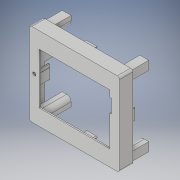
# Autodesk Inventor part: case_top
Saved by Autodesk Inventor 2019 (Build 230136000, 136)
## iProperties
Created: 2019-03-26
Part Number: case_top
Material: Generic
Document SubType Name: Modeling
Designer: janza
Density: 1 g/cm^3
Appearance: Default
Author: janza
## iProperties of the stored document case_top_3DPrint.ipt
Created: 2019-03-30
Part Number: case_top_3DPrint
Material: Generic
Document SubType Name: Modeling
Designer: janza
Density: 1 g/cm^3
Appearance: Default
Author: janza
Autodesk Inventor part; units mm, degrees
ref_plane "YZ Plane" through (0, 0, 0) normal (1, 0, 0) x (0, 1, 0)
ref_plane "XZ Plane" through (0, 0, 0) normal (0, 1, 0) x (-1, 0, 0)
ref_plane "XY Plane" through (0, 0, 0) normal (0, 0, 1) x (1, 0, 0)
sketch "vrsek" plane through (0, 0, 0) normal (0, 0, 1) x (1, 0, 0)
  line L0 (0, 0) -> (78.5, 0)
  line L1 (78.5, 0) -> (78.5, 72)
  line L2 (78.5, 72) -> (0, 72)
  line L3 (0, 72) -> (0, 0)
  dimension "d0" = 78.5
  dimension "d1" = 72
  constraints: 8 end point, 2 parallel, 1 horizontal, 1 perpendicular
  measures "d0" distance of L2.end L1.end
  measures "d1" distance of L1.end L0.end
extrude "Extrusion1" add sketch "vrsek" along normal blind 1.2 and the other way blind 0.4
sketch "displej_vyrez" plane through (0, 0, 1.2) normal (0, 0, 1) x (1, 0, 0)
  line L0 (0, 72) -> (0, 0) projected
  line L1 (78.5, 0) -> (78.5, 72) projected
  line L2 (0, 36) -> (7, 36)
  line L3 (7, 36) -> (7, 59.15)
  line L4 (7, 59.15) -> (71.2, 59.15)
  line L5 (71.2, 59.15) -> (71.2, 53.35)
  line L6 (71.2, 53.35) -> (72.7, 53.35)
  line L7 (72.7, 53.35) -> (72.7, 40.95)
  line L8 (72.7, 40.95) -> (71.2, 40.95)
  line L9 (7, 36) -> (7, 12.85)
  line L10 (7, 12.85) -> (71.2, 12.85)
  line L11 (71.2, 12.85) -> (71.2, 40.95)
  line L12 (0, 0) -> (78.5, 0) projected
  dimension "d4" = 7
  dimension "d5" = 23.15
  dimension "d6" = 64.2
  dimension "d7" = 5.8
  dimension "d8" = 1.5
  dimension "d9" = 12.4
  dimension "d10" = 1.5
  dimension "d11" = 23.15
  dimension "d12" = 36
  constraints: 20 end point, 6 perpendicular, 1 horizontal, 1 midpoint, 1 parallel, 1 point on line, 1 vertical
  measures "d4" distance of L2.start L2.end
  measures "d5" distance of L2.end L3.end
  measures "d6" distance of L3.end L4.end
  measures "d7" distance of L4.end L5.end
  measures "d8" distance of L5.end L6.end
  measures "d9" distance of L6.end L7.end
  measures "d10" distance of L7.end L8.end
  measures "d11" distance of L2.end L9.end
  measures "d12" distance between parallel lines of L12 L2
extrude "Extrusion2" cut sketch "displej_vyrez" against normal blind 3
sketch "resetTL_zarez_vedeni" plane through (0, 0, 1.2) normal (0, 0, 1) x (1, 0, 0)
  line L0 (0.5, 40.85) -> (5, 40.85)
  line L1 (5, 40.85) -> (5, 33.85)
  line L2 (5, 33.85) -> (0.5, 33.85)
  line L3 (0.5, 33.85) -> (0.5, 40.85)
  line L4 (0, 0) -> (78.5, 0) projected
  line L5 (7, 12.85) -> (7, 59.15) projected
  line L6 (71.2, 12.85) -> (7, 12.85) projected
  dimension "d15" = 4.5
  dimension "d16" = 7
  dimension "d19" = 2
  dimension "d20" = 21
  constraints: 8 end point, 2 parallel, 1 horizontal, 1 perpendicular
  measures "d15" distance of L1.end L2.end
  measures "d16" distance of L0.end L1.end
  measures "d19" distance between parallel lines of L5 L1
  measures "d20" distance between parallel lines of L6 L2
sketch "resetTL_vnitrek_vybrani" plane through (0, 0, -0.4) normal (0, 0, -1) x (-1, 0, 0)
  line L0 (-5, 33.85) -> (-0.8, 33.85)
  line L1 (-5, 40.85) -> (-5, 33.85)
  line L2 (-0.8, 40.85) -> (-5, 40.85)
  line L3 (-0.8, 33.85) -> (-0.8, 40.85)
  line L4 (0, 0) -> (0, 72) projected
  line L5 (0, 72) -> (0, 0) projected
  line L6 (0, 72) -> (-78.5, 72) projected
  point P0 (-0.8, 37.35)
  dimension "d106" = 31.15
  dimension "d107" = 4.2
  dimension "d108" = 7
  dimension "d109" = 0.8
  constraints: 8 end point, 1 midpoint
  measures "d106" distance between parallel lines of L6 L2
  measures "d107" distance of L2.start L1.start
  measures "d108" distance of L1.start L0.start
  measures "d109" distance between parallel lines of L4 L3
extrude "Extrusion3" cut sketch "resetTL_vnitrek_vybrani" against normal blind 0.9
sketch "resetTL_dira" plane through (0, 0, 0.5) normal (0, 0, -1) x (-1, 0, 0)
  line L0 (-5, 33.85) -> (-5, 40.85)
  circle A0 centre (-2.743122, 37.35) radius 1.5
  point P0 (0, 0)
  dimension "d23" = 3
  constraints: 1 centre point
  measures "d23" diameter of A0
extrude "Extrusion4" cut sketch "resetTL_dira" against normal blind 2
sketch "spojeni_srouby" plane through (0, 0, -0.4) normal (0, 0, -1) x (-1, 0, 0)
  line L0 (-8, 68) -> (-8, 72)
  line L1 (-4, 72) -> (0, 72)
  line L2 (-8, 72) -> (0, 72)
  line L3 (0, 72) -> (0, 71.785113)
  line L4 (0, 72) -> (0, 0)
  line L5 (0, 0) -> (0, 36)
  line L6 (-8, 4) -> (-8, 0)
  line L7 (-4, 0) -> (0, 0)
  line L8 (-8, 0) -> (0, 0)
  line L9 (0, 0) -> (0, 0.214887)
  line L10 (0, 0) -> (0, 72)
  line L11 (-70.5, 68) -> (-70.5, 72)
  line L12 (-74.5, 72) -> (-78.5, 72)
  line L13 (-70.5, 72) -> (-78.5, 72)
  line L14 (-78.5, 72) -> (-78.5, 71.785113)
  line L15 (-70.5, 4) -> (-70.5, 0)
  line L16 (-74.5, 0) -> (-78.5, 0)
  line L17 (-70.5, 0) -> (-78.5, 0)
  line L18 (-78.5, 0) -> (-78.5, 0.214887)
  line L19 (-78.5, 72) -> (-78.5, 72)
  line L20 (-78.5, 0) -> (-78.5, 0)
  line L21 (-78.5, 0) -> (-70.5, 0)
  line L22 (-74.5, 64) -> (-78.5, 64)
  line L23 (-78.5, 64) -> (-78.5, 72)
  arc A0 (-74.5, 64) -> (-70.5, 68) centre (-74.5, 68) ccw
  line L24 (-74.5, 8) -> (-78.5, 8)
  arc A1 (-70.5, 4) -> (-74.5, 8) centre (-74.5, 4) ccw
  line L25 (-4, 8) -> (0, 8)
  arc A2 (-4, 8) -> (-8, 4) centre (-4, 4) ccw
  line L26 (-4, 64) -> (0, 64)
  arc A3 (-8, 68) -> (-4, 64) centre (-4, 68) ccw
  line L27 (0, 72) -> (0, 56.55)
  line L28 (0, 72) -> (0, 64)
  line L29 (0, 8) -> (0, 0)
  line L30 (-78.5, 0) -> (-78.5, 8)
  line L31 (-78.5, 64) -> (-78.5, 72)
  line L32 (-70.5, 72) -> (-78.5, 72)
  line L33 (0, 72) -> (-8, 72)
  constraints: 68 end point, 8 point on circle, 5 perpendicular, 4 centre point, 4 tangent, 3 collinear, 2 point on line, 2 vertical, 1 midpoint
extrude "Extrusion7" add sketch "spojeni_srouby" along normal blind 26.5
sketch "diry_zavitova_vlozka" plane through (0, 0, -26.9) normal (0, 0, -1) x (-1, 0, 0)
  arc A0 (-70.5, 4) -> (-74.5, 8) centre (-74.5, 4) ccw projected
  arc A1 (-4, 8) -> (-8, 4) centre (-4, 4) ccw projected
  arc A2 (-8, 68) -> (-4, 64) centre (-4, 68) ccw projected
  arc A3 (-74.5, 64) -> (-70.5, 68) centre (-74.5, 68) ccw projected
  point P0 (0, 0)
  constraints: 4 coincident
hole "Hole1" at (74.5, 4, -26.9) at (4, 4, -26.9) at (4, 68, -26.9) at (74.5, 68, -26.9) direction (0, 0, 1) diameter 3.3 depth 12 countersink diameter 3.75 countersink angle 10
sketch "Sketch10" plane through (0, 0, -0.4) normal (0, 0, -1) x (-1, 0, 0)
  line L0 (-71.2, 59.15) -> (-7, 59.15) projected
  line L1 (-7, 59.15) -> (-7, 12.85) projected
  line L2 (-7, 12.85) -> (-71.2, 12.85) projected
  line L3 (-71.2, 12.85) -> (-71.2, 40.95) projected
  line L4 (-71.2, 40.95) -> (-72.7, 40.95) projected
  line L5 (-72.7, 40.95) -> (-72.7, 53.35) projected
  line L6 (-72.7, 53.35) -> (-71.2, 53.35) projected
  line L7 (-70.5, 0) -> (-8, 0) projected
  line L8 (-8, 0) -> (-8, 4) projected
  arc A0 (-4, 8) -> (-8, 4) centre (-4, 4) ccw projected
  line L9 (-4, 8) -> (0, 8) projected
  line L10 (0, 8) -> (0, 64) projected
  line L11 (0, 64) -> (-4, 64) projected
  arc A1 (-8, 68) -> (-4, 64) centre (-4, 68) ccw projected
  line L12 (-8, 68) -> (-8, 72) projected
  line L13 (-8, 72) -> (-70.5, 72) projected
  line L14 (-78.5, 64) -> (-78.5, 8) projected
  line L15 (-0.8, 40.85) -> (-0.8, 33.85) projected
  line L16 (-0.8, 33.85) -> (-5, 33.85) projected
  line L17 (-5, 33.85) -> (-5, 40.85) projected
  line L18 (-5, 40.85) -> (-0.8, 40.85) projected
  line L19 (-7, 12.85) -> (-71.2, 12.85) projected
  line L20 (-71.2, 12.85) -> (-71.2, 40.95) projected
  line L21 (-71.2, 40.95) -> (-72.7, 40.95) projected
  line L22 (-72.7, 40.95) -> (-72.7, 53.35) projected
  line L23 (-72.7, 53.35) -> (-71.2, 53.35) projected
  line L24 (-71.2, 53.35) -> (-71.2, 59.15) projected
  line L25 (-71.2, 59.15) -> (-7, 59.15) projected
  line L26 (-7, 59.15) -> (-7, 12.85) projected
  line L27 (-73.7, 61.65) -> (-73.7, 55.85)
  line L28 (-73.7, 55.85) -> (-75.2, 55.85)
  line L29 (-75.2, 55.85) -> (-75.2, 38.45)
  line L30 (-75.2, 38.45) -> (-73.7, 38.45)
  line L31 (-73.7, 38.45) -> (-73.7, 10.35)
  line L32 (-73.7, 10.35) -> (-4.5, 10.35)
  line L33 (-4.5, 10.35) -> (-4.5, 61.65)
  line L34 (-4.5, 61.65) -> (-73.7, 61.65)
  line L35 (-70.5, 4) -> (-70.5, 0) projected
  line L36 (-70.5, 72) -> (-70.5, 68) projected
  arc A2 (-74.5, 64) -> (-70.5, 68) centre (-74.5, 68) ccw projected
  line L37 (-74.5, 64) -> (-78.5, 64) projected
  line L38 (-78.5, 8) -> (-74.5, 8) projected
  arc A3 (-70.5, 4) -> (-74.5, 8) centre (-74.5, 4) ccw projected
  point P0 (0, 0)
  dimension "d58" = 2.5
  constraints: 16 end point, 7 other
  measures "d58" distance between parallel lines of L24 L27
extrude "Extrusion8" cut sketch "Sketch10" against normal blind 0.4 contours L33 L16 L17 L18 | L18 L17 L16 L33 L32 L31 L30 L29 L28 L27 L34
sketch "dira_RJ45" plane through (0, 0, -0.4) normal (0, 0, -1) x (-1, 0, 0)
  line L0 (1.6, 39.75) -> (0, 39.75)
  line L1 (0, 39.75) -> (0, 56.55)
  line L2 (0, 56.55) -> (1.6, 56.55)
  line L3 (1.6, 56.55) -> (1.6, 39.75)
  line L4 (-70.5, 0) -> (-8, 0) projected
  line L5 (0, 8) -> (0, 64) projected
  line L6 (0, 72) -> (-8, 72) projected
  point P0 (0, 0)
  point P1 (-78.5, 0)
  dimension "d61" = 1.6
  dimension "d62" = 16.8
  dimension "d64" = 0
  dimension "d74" = 15.45
  constraints: 8 end point, 2 parallel, 1 horizontal, 1 perpendicular
  measures "d61" distance of L1.end L2.end
  measures "d62" distance of L0.end L1.end
  measures "d64" distance between parallel lines of L5 L1
  measures "d74" distance between parallel lines of L6 L2
extrude "Extrusion9" add sketch "dira_RJ45" along normal blind 17.3 and the other way blind 1.6
sketch "Sketch12" plane through (0, 0, -0.4) normal (0, 0, -1) x (-1, 0, 0)
  line L0 (0, 56.55) -> (0, 64) projected
  line L1 (0, 64) -> (0, 72) projected
  line L2 (0, 72) -> (-8, 72) projected
  line L3 (-8, 72) -> (-70.5, 72) projected
  line L4 (-70.5, 72) -> (-78.5, 72) projected
  line L5 (-78.5, 72) -> (-78.5, 64) projected
  line L6 (-78.5, 64) -> (-78.5, 8) projected
  line L7 (-92, 8) -> (-92, 0) projected
  line L8 (-78.5, 0) -> (-70.5, 0) projected
  line L9 (-70.5, 0) -> (-8, 0) projected
  line L10 (-8, 0) -> (0, 0) projected
  line L11 (0, 0) -> (0, 8) projected
  line L12 (0, 8) -> (0, 39.75) projected
  line L13 (1.6, 56.55) -> (1.6, 63)
  line L14 (1.6, 63) -> (1.6, 73.6)
  line L15 (1.6, 73.6) -> (-8, 73.6)
  line L16 (-8, 73.6) -> (-80.1, 73.6)
  line L17 (-80.1, 73.6) -> (-80.1, 64)
  line L18 (-80.1, 64) -> (-80.1, 8)
  line L19 (-80.1, -1.6) -> (-8, -1.6)
  line L20 (-8, -1.6) -> (1.6, -1.6)
  line L21 (1.6, -1.6) -> (1.6, 7)
  line L22 (1.6, 7) -> (1.6, 39.75)
  line L23 (1.6, 56.55) -> (0, 56.55) projected
  line L24 (0, 56.55) -> (1.6, 56.55)
  line L25 (0, 39.75) -> (0, 56.55) projected
  line L26 (1.6, 39.75) -> (0, 39.75)
  line L27 (-80.1, 8) -> (-80.1, -1.6)
  constraints: 26 end point, 1 collinear, 1 horizontal, 1 perpendicular, 5 other
sketch "Sketch12 outline for Extrusion10" plane through (0, 0, -0.4) normal (0, 0, -1) x (-1, 0, 0)
  line L0 (0, 8) -> (0, 0)
  line L1 (0, 39.75) -> (0, 8)
  line L2 (1.6, 39.75) -> (0, 39.75)
  line L3 (1.6, 7) -> (1.6, 39.75)
  line L4 (1.6, -1.6) -> (1.6, 7)
  line L5 (-8, -1.6) -> (1.6, -1.6)
  line L6 (-80.1, -1.6) -> (-8, -1.6)
  line L7 (-80.1, 8) -> (-80.1, -1.6)
  line L8 (-80.1, 64) -> (-80.1, 8)
  line L9 (-80.1, 73.6) -> (-80.1, 64)
  line L10 (-8, 73.6) -> (-80.1, 73.6)
  line L11 (1.6, 73.6) -> (-8, 73.6)
  line L12 (1.6, 63) -> (1.6, 73.6)
  line L13 (1.6, 56.55) -> (1.6, 63)
  line L14 (0, 56.55) -> (1.6, 56.55)
  line L15 (0, 64) -> (0, 56.55)
  line L16 (0, 72) -> (0, 64)
  line L17 (-8, 72) -> (0, 72)
  line L18 (-70.5, 72) -> (-8, 72)
  line L19 (-78.5, 72) -> (-70.5, 72)
  line L20 (-78.5, 64) -> (-78.5, 72)
  line L21 (-78.5, 8) -> (-78.5, 64)
  line L22 (-78.5, 0) -> (-78.5, 8)
  line L23 (-70.5, 0) -> (-78.5, 0)
  line L24 (-8, 0) -> (-70.5, 0)
  line L25 (0, 0) -> (-8, 0)
extrude "Extrusion10" add sketch "Sketch12 outline for Extrusion10" along normal blind 10.5 and the other way blind 1.6
fillet "Fillet1" radius 2 4 edges at (-1.6, 73.6, -4.85) (-1.6, -1.6, -4.85) (80.1, 73.6, -4.85) (80.1, -1.6, -4.85)
sketch "Sketch13" plane through (0, 0, -0.4) normal (0, 0, -1) x (-1, 0, 0)
  line L0 (-1.2, 33.75) -> (-1.2, 24.65)
  line L1 (-0.4, 23.85) -> (0, 23.85)
  line L2 (0, 23.85) -> (0, 36.75)
  line L3 (0, 8) -> (0, 64) projected
  line L4 (0, 36.75) -> (-0.4, 36.75)
  line L5 (-0.8, 36.35) -> (-0.8, 33.95)
  line L6 (-0.8, 33.85) -> (-4.5, 33.85) projected
  line L7 (-0.9, 33.85) -> (-1.1, 33.85)
  arc A0 (-0.4, 36.75) -> (-0.8, 36.35) centre (-0.4, 36.35) ccw
  line L8 (-35.05, 1.2) -> (-43.45, 1.2)
  line L9 (-44.25, 0.4) -> (-44.25, 0)
  line L10 (-44.25, 0) -> (-34.25, 0)
  line L11 (-34.25, 0) -> (-34.25, 0.4)
  line L12 (-70.5, 0) -> (-8, 0) projected
  arc A1 (-1.2, 24.65) -> (-0.4, 23.85) centre (-0.4, 24.65) ccw
  line L13 (-34.25, 72) -> (-44.25, 72)
  line L14 (-44.25, 72) -> (-44.25, 71.6)
  line L15 (-43.45, 70.8) -> (-35.05, 70.8)
  line L16 (-34.25, 71.6) -> (-34.25, 72)
  line L17 (-8, 72) -> (-70.5, 72) projected
  line L18 (-78.1, 41) -> (-78.5, 41)
  line L19 (-78.5, 41) -> (-78.5, 31)
  line L20 (-78.5, 31) -> (-78.1, 31)
  line L21 (-77.3, 31.8) -> (-77.3, 40.2)
  line L22 (-78.5, 64) -> (-78.5, 8) projected
  arc A2 (-78.1, 31) -> (-77.3, 31.8) centre (-78.1, 31.8) ccw
  arc A3 (-77.3, 40.2) -> (-78.1, 41) centre (-78.1, 40.2) ccw
  arc A4 (-43.45, 1.2) -> (-44.25, 0.4) centre (-43.45, 0.4) ccw
  arc A5 (-34.25, 0.4) -> (-35.05, 1.2) centre (-35.05, 0.4) ccw
  arc A6 (-44.25, 71.6) -> (-43.45, 70.8) centre (-43.45, 71.6) ccw
  arc A7 (-35.05, 70.8) -> (-34.25, 71.6) centre (-35.05, 71.6) ccw
  line L23 (-0.8, 33.95) -> (-0.8, 33.85)
  line L24 (-0.8, 33.85) -> (-1.2, 33.85)
  line L25 (-1.2, 33.85) -> (-1.2, 33.75)
  point P0 (0, 0)
  point P1 (-1.2, 23.85)
  point P2 (0, 39.75)
  point P3 (-0.8, 36.75)
  point P4 (-44.25, 1.2)
  point P5 (-39.25, 1.2)
  point P6 (-39.25, 0)
  point P7 (-44.25, 70.8)
  point P8 (-34.25, 70.8)
  point P9 (-39.25, 72)
  point P10 (-39.25, 72)
  point P11 (-77.3, 31)
  point P12 (-78.5, 36)
  point P13 (-78.5, 36)
  dimension "d76" = 1.2
  dimension "d77" = 10
  dimension "d79" = 0
  dimension "d80" = 0.8
  dimension "d81" = 0.4
  dimension "d82" = 10
  dimension "d83" = 1.2
  dimension "d84" = 0
  dimension "d86" = 0
  dimension "d87" = 0.8
  dimension "d89" = 10
  dimension "d90" = 1.2
  dimension "d91" = 0
  dimension "d92" = 0
  dimension "d93" = 1.2
  dimension "d94" = 10
  dimension "d95" = 0
  dimension "d96" = 0
  dimension "d97" = 0.8
  constraints: 42 end point, 17 point on line, 16 point on circle, 16 tangent, 8 centre point, 7 parallel, 6 midpoint, 6 perpendicular, 5 equal radius, 4 horizontal, 1 collinear, 1 vertical
  measures "d76" distance of L1.end point (-1.2, 23.85)
  measures "d77" distance of point (-1.2, 23.85) L24.end
  measures "d79" distance between parallel lines of L3 L2
  measures "d80" distance of L2.end point (-0.8, 36.75)
  measures "d81" radius of A0
  measures "d82" distance of L10.end L9.end
  measures "d83" distance of L9.end point (-44.25, 1.2)
  measures "d84" distance between parallel lines of L12 L10
  measures "d86" horizontal distance of point (-39.25, 0) point (-39.25, 1.2)
  measures "d87" radius of A1
  measures "d89" distance of point (-34.25, 70.8) point (-44.25, 70.8)
  measures "d90" distance of point (-44.25, 70.8) L13.end
  measures "d91" distance of point (-39.25, 72) point (-39.25, 72)
  measures "d92" distance between parallel lines of L17 L13
  measures "d93" distance of point (-77.3, 31) L19.end
  measures "d94" distance of L19.end L18.end
  measures "d95" distance of point (-78.5, 36) point (-78.5, 36)
  measures "d96" distance between parallel lines of L22 L19
  measures "d97" radius of A2
extrude "Extrusion11" add sketch "Sketch13" along normal blind 14 and the other way blind 1
body "Solid1"
